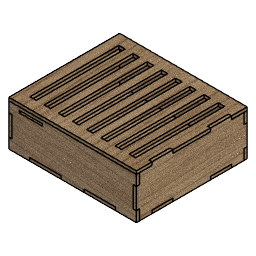
CAJA MADERA (Autodesk Fusion 360 design; units mm, degrees)
part number: 2026-06-24-23-30-10-522
part number: 2026-06-24-23-30-19-189
Autodesk Fusion 360 part; units mm, degrees
sketch "Boceto1" plane through (0, 0, 0) normal (0, 0, 1) x (1, 0, 0) in component "caja"
  line L0 (0, 0) -> (122, 0)
  line L1 (122, 0) -> (122, 106)
  line L2 (122, 106) -> (0, 106)
  line L3 (0, 106) -> (0, 0)
  dimension "d1" = 122
  dimension "d2" = 106
  constraint horizontal L0
  constraint vertical L1
  constraint horizontal L2
  constraint vertical L3
  constraint coincident L0.start L3.end
  measures "d1" distance of L0.start L0.end
  measures "d2" distance of L0.start L2.end
extrude "Extruir1" add sketch "Boceto1" along normal blind 3 makes body 1 in component "caja"
sketch "Boceto2" plane through (0, 0, 0) normal (0, -1, 0) x (1, 0, 0) in component "caja"
  line L0 (0, 0) -> (122, 0)
  line L1 (122, 0) -> (122, 3)
  line L2 (122, 3) -> (0, 3)
  line L3 (0, 3) -> (0, 0)
  line L4 (0, 0) -> (122, 0)
  line L5 (122, 0) -> (122, 40)
  line L6 (122, 40) -> (0, 40)
  line L7 (0, 40) -> (0, 0)
  line L8 (20, 0) -> (50, 0)
  line L9 (50, 0) -> (50, 3)
  line L10 (50, 3) -> (20, 3)
  line L11 (20, 3) -> (20, 0)
  line L12 (102, 0) -> (72, 0)
  line L13 (72, 0) -> (72, 3)
  line L14 (72, 3) -> (102, 3)
  line L15 (102, 3) -> (102, 0)
  line L16 (122, 30) -> (119, 30)
  line L17 (119, 30) -> (119, 10)
  line L18 (119, 10) -> (122, 10)
  line L19 (122, 10) -> (122, 30)
  line L20 (0, 30) -> (3, 30)
  line L21 (3, 30) -> (3, 10)
  line L22 (3, 10) -> (0, 10)
  line L23 (0, 10) -> (0, 30)
  point P0 (122, 20)
  point P1 (0, 20)
  dimension "d5" = 122
  dimension "d6" = 40
  dimension "d13" = 30
  dimension "d14" = 3
  dimension "d15" = 20
  dimension "d16" = 30
  dimension "d17" = 3
  dimension "d18" = 20
  dimension "d19" = 3
  dimension "d20" = 20
  dimension "d21" = 3
  dimension "d22" = 20
  constraint horizontal L4
  constraint vertical L5
  constraint horizontal L6
  constraint vertical L7
  constraint coincident L0.start L3.end
  constraint horizontal L8
  constraint vertical L9
  constraint horizontal L10
  constraint vertical L11
  constraint coincident L4 L8.start
  constraint horizontal L12
  constraint vertical L13
  constraint horizontal L14
  constraint vertical L15
  constraint coincident L4 L12.start
  constraint horizontal L16
  constraint vertical L17
  constraint horizontal L18
  constraint vertical L19
  constraint coincident L5 L16.start
  constraint midpoint L5 P0
  constraint midpoint L19 P0
  constraint horizontal L20
  constraint vertical L21
  constraint horizontal L22
  constraint vertical L23
  constraint coincident L7 L20.start
  constraint midpoint L7 P1
  constraint midpoint L23 P1
  measures "d5" distance of L0.start L0.end
  measures "d6" distance of L0.start L6.end
  measures "d13" distance of L8.start L8.end
  measures "d14" distance of L8.start L10.end
  measures "d15" distance of L0.start L8.start
  measures "d16" distance of L12.start L12.end
  measures "d17" distance of L12.start L14.end
  measures "d18" distance of L0.end L12.start
  measures "d19" distance of L16.start L16.end
  measures "d20" distance of L16.start L18.end
  measures "d21" distance of L20.start L20.end
  measures "d22" distance of L20.start L22.end
extrude "Extruir2" add sketch "Boceto2" against normal blind 3 separate body makes body 2 in component "caja"
sketch "Boceto3" plane through (122, 0, 0) normal (1, 0, 0) x (0, 1, 0) in component "caja"
  line L0 (0, 0) -> (106, 0)
  line L1 (106, 0) -> (106, 3)
  line L2 (106, 3) -> (0, 3)
  line L3 (0, 3) -> (0, 0)
  line L4 (0, 0) -> (106, 0)
  line L5 (106, 0) -> (106, 40)
  line L6 (106, 40) -> (0, 40)
  line L7 (0, 40) -> (0, 0)
  line L8 (15, 0) -> (35, 0)
  line L9 (35, 0) -> (35, 3)
  line L10 (35, 3) -> (15, 3)
  line L11 (15, 3) -> (15, 0)
  line L12 (91, 0) -> (71, 0)
  line L13 (71, 0) -> (71, 3)
  line L14 (71, 3) -> (91, 3)
  line L15 (91, 3) -> (91, 0)
  line L16 (15, 40) -> (35, 40)
  line L17 (35, 40) -> (35, 43)
  line L18 (35, 43) -> (15, 43)
  line L19 (15, 43) -> (15, 40)
  line L20 (71, 40) -> (91, 40)
  line L21 (91, 40) -> (91, 43)
  line L22 (91, 43) -> (71, 43)
  line L23 (71, 43) -> (71, 40)
  dimension "d9" = 106
  dimension "d10" = 40
  dimension "d25" = 20
  dimension "d26" = 3
  dimension "d27" = 15
  dimension "d28" = 20
  dimension "d29" = 3
  dimension "d30" = 15
  dimension "d45" = 20
  dimension "d46" = 3
  dimension "d47" = 20
  dimension "d48" = 3
  constraint horizontal L4
  constraint vertical L5
  constraint horizontal L6
  constraint vertical L7
  constraint coincident L0.start L3.end
  constraint horizontal L8
  constraint vertical L9
  constraint horizontal L10
  constraint vertical L11
  constraint coincident L0 L8.start
  constraint horizontal L12
  constraint vertical L13
  constraint horizontal L14
  constraint vertical L15
  constraint coincident L4 L12.start
  constraint horizontal L16
  constraint vertical L17
  constraint horizontal L18
  constraint vertical L19
  constraint coincident L6 L16.start
  constraint horizontal L20
  constraint vertical L21
  constraint horizontal L22
  constraint vertical L23
  constraint coincident L6 L20.start
  measures "d9" distance of L0.start L0.end
  measures "d10" distance of L0.start L6.end
  measures "d25" distance of L8.start L8.end
  measures "d26" distance of L8.start L10.end
  measures "d27" distance of L0.start L8.start
  measures "d28" distance of L12.start L12.end
  measures "d29" distance of L12.start L14.end
  measures "d30" distance of L0.end L12.start
  measures "d45" distance of L16.start L16.end
  measures "d46" distance of L16.start L18.end
  measures "d47" distance of L20.start L20.end
  measures "d48" distance of L20.start L22.end
extrude "Extruir3" add sketch "Boceto3" against normal blind 3 separate body contours L0 L2 L3 L4 L7 L11 | L0 L2 L4 L8 L9 L10 L11 | L2 L5 L6 L7 L10 L14 L16 L20 | L0 L2 L4 L9 L13 | L0 L2 L4 L12 L13 L14 L15 | L0 L1 L2 L4 L5 L15 makes body 3 in component "caja"
extrude "Extruir4" cut sketch "Boceto2" against normal blind 3 contours L0 L2 L4 L8 L9 L10 L11 | L7 L20 L21 L22 L23 | L0 L2 L4 L12 L13 L14 L15 | L5 L16 L17 L18 L19 bodies 2 in component "caja"
extrude "Extruir5" cut sketch "Boceto3" against normal blind 3 contours L0 L2 L4 L8 L9 L10 L11 | L0 L2 L4 L12 L13 L14 L15 bodies 3 in component "caja"
copy_body "CopiarPegarCuerpos1" bodies 2 makes body 4 in component "caja"
move_body "Desplazar1" bodies 4 to x (1, 0, 0) y (0, 1, 0) z (0, 0, 1) at (0, 126, 0) in component "caja"
copy_body "CopiarPegarCuerpos2" bodies 3 makes body 5 in component "caja"
move_body "Desplazar2" bodies 5 to x (1, 0, 0) y (0, 1, 0) z (0, 0, 1) at (-138, 0, 0) in component "caja"
move_body "Alinear1" bodies 5 to x (1, 0, 0) y (0, 1, 0) z (0, 0, 1) at (19, 0, 0) in component "caja"
move_body "Alinear2" bodies 4 to x (1, 0, 0) y (0, 1, 0) z (0, 0, 1) at (0, -23, 0) in component "caja"
combine "Combinar1" operation cut target body 1 tool bodies 2 5 4 3 keep tools in component "caja"
combine "Combinar2" operation cut target body 5 tool bodies 4 2 keep tools in component "caja"
combine "Combinar3" operation cut target body 3 tool bodies 2 4 keep tools in component "caja"
sketch "Boceto4" plane through (0, 0, 0) normal (0, -1, 0) x (1, 0, 0) in component "caja"
  line L0 (50, 3) -> (50, 0)
  line L1 (50, 0) -> (72, 0)
  line L2 (72, 0) -> (72, 3)
  line L3 (72, 3) -> (102, 3)
  line L4 (102, 3) -> (102, 0)
  line L5 (102, 0) -> (122, 0)
  line L6 (122, 0) -> (122, 10)
  line L7 (122, 10) -> (119, 10)
  line L8 (119, 10) -> (119, 30)
  line L9 (119, 30) -> (122, 30)
  line L10 (122, 30) -> (122, 40)
  line L11 (122, 40) -> (0, 40)
  line L12 (0, 40) -> (0, 30)
  line L13 (0, 30) -> (3, 30)
  line L14 (3, 30) -> (3, 10)
  line L15 (3, 10) -> (0, 10)
  line L16 (0, 10) -> (0, 0)
  line L17 (0, 0) -> (20, 0)
  line L18 (20, 0) -> (20, 3)
  line L19 (20, 3) -> (50, 3)
  line L20 (10.0905, 37.0618) -> (32.0905, 37.0618)
  line L21 (32.0905, 37.0618) -> (32.0905, 35.0618)
  line L22 (32.0905, 35.0618) -> (10.0905, 35.0618)
  line L23 (10.0905, 35.0618) -> (10.0905, 37.0618)
  dimension "d33" = 22
  dimension "d34" = 2
  constraint horizontal L20
  constraint vertical L21
  constraint horizontal L22
  constraint vertical L23
  measures "d33" distance of L20.start L20.end
  measures "d34" distance of L20.start L22.end
extrude "Extruir6" cut sketch "Boceto4" against normal blind 3 contours L20 L21 L22 L23 bodies 2 in component "caja"
sketch "Boceto5" plane through (0, 0, 0) normal (-1, 0, 0) x (0, -1, 0) in component "caja"
  line L0 (-3, 0) -> (-3, 10)
  line L1 (-3, 10) -> (0, 10)
  line L2 (0, 10) -> (0, 30)
  line L3 (0, 30) -> (-3, 30)
  line L4 (-3, 30) -> (-3, 40)
  line L5 (-3, 40) -> (-103, 40)
  line L6 (-103, 40) -> (-103, 30)
  line L7 (-103, 30) -> (-106, 30)
  line L8 (-106, 30) -> (-106, 10)
  line L9 (-106, 10) -> (-103, 10)
  line L10 (-103, 10) -> (-103, 0)
  line L11 (-103, 0) -> (-91, 0)
  line L12 (-91, 0) -> (-91, 3)
  line L13 (-91, 3) -> (-71, 3)
  line L14 (-71, 3) -> (-71, 0)
  line L15 (-71, 0) -> (-35, 0)
  line L16 (-35, 0) -> (-35, 3)
  line L17 (-35, 3) -> (-15, 3)
  line L18 (-15, 3) -> (-15, 0)
  line L19 (-15, 0) -> (-3, 0)
  line L20 (-12.0898, 37.3242) -> (-7.0898, 37.3242)
  line L21 (-7.0898, 37.3242) -> (-7.0898, 32.3242)
  line L22 (-7.0898, 32.3242) -> (-12.0898, 32.3242)
  line L23 (-12.0898, 32.3242) -> (-12.0898, 37.3242)
  dimension "d37" = 5
  dimension "d38" = 5
  constraint horizontal L20
  constraint vertical L21
  constraint horizontal L22
  constraint vertical L23
  measures "d37" distance of L20.start L20.end
  measures "d38" distance of L20.start L22.end
extrude "Extruir7" cut sketch "Boceto5" against normal blind 3 contours L20 L21 L22 L23 bodies 5 in component "caja"
sketch "Boceto8" plane through (0, 0, 40) normal (0, 0, 1) x (-1, 0, 0) in component "caja"
  line L0 (0, -103) -> (-122, -103)
  line L1 (-122, -103) -> (-122, -106)
  line L2 (-122, -106) -> (0, -106)
  line L3 (0, -106) -> (0, -103)
  line L4 (0, -106) -> (-122, -106)
  line L5 (-122, -106) -> (-122, 0)
  line L6 (-122, 0) -> (0, 0)
  line L7 (0, 0) -> (0, -106)
  line L8 (-10.0686, -95.2773) -> (-15.0686, -95.2773)
  line L9 (-15.0686, -95.2773) -> (-15.0686, -15.2773)
  line L10 (-15.0686, -15.2773) -> (-10.0686, -15.2773)
  line L11 (-10.0686, -15.2773) -> (-10.0686, -95.2773)
  dimension "d41" = 122
  dimension "d42" = 106
  dimension "d51" = 5
  dimension "d52" = 80
  constraint horizontal L4
  constraint vertical L5
  constraint horizontal L6
  constraint vertical L7
  constraint coincident L2.end L3.start
  constraint horizontal L8
  constraint vertical L9
  constraint horizontal L10
  constraint vertical L11
  measures "d41" distance of L2.end L1.end
  measures "d42" distance of L2.end L6.end
  measures "d51" distance of L8.start L8.end
  measures "d52" distance of L8.start L10.end
extrude "Extruir8" add sketch "Boceto8" along normal blind 3 separate body contours L0 L1 L2 L3 L4 L5 L7 | L0 L5 L6 L7 | L8 L9 L10 L11 makes body 6 in component "caja"
extrude "Extruir9" add sketch "Boceto3" against normal blind 3 contours L6 L16 L17 L18 L19 | L6 L20 L21 L22 L23 bodies 3 in component "caja"
combine "Combinar4" operation cut target body 6 tool bodies 3 keep tools in component "caja"
sketch "Boceto9" plane through (0, 0, 43) normal (0, 0, 1) x (-1, 0, 0) in component "caja"
  line L0 (-119, -91) -> (-122, -91)
  line L1 (-122, -91) -> (-122, -106)
  line L2 (-122, -106) -> (0, -106)
  line L3 (0, -106) -> (0, 0)
  line L4 (0, 0) -> (-122, 0)
  line L5 (-122, 0) -> (-122, -15)
  line L6 (-122, -15) -> (-119, -15)
  line L7 (-119, -15) -> (-119, -35)
  line L8 (-119, -35) -> (-122, -35)
  line L9 (-122, -35) -> (-122, -71)
  line L10 (-122, -71) -> (-119, -71)
  line L11 (-119, -71) -> (-119, -91)
  line L12 (-9.7376, -95.5293) -> (-15.7376, -95.5293)
  line L13 (-15.7376, -95.5293) -> (-15.7376, -10.5293)
  line L14 (-15.7376, -10.5293) -> (-9.7376, -10.5293)
  line L15 (-9.7376, -10.5293) -> (-9.7376, -95.5293)
  dimension "d53" = 6
  dimension "d54" = 85
  constraint horizontal L12
  constraint vertical L13
  constraint horizontal L14
  constraint vertical L15
  measures "d53" distance of L12.start L12.end
  measures "d54" distance of L12.start L14.end
extrude "Extruir10" cut sketch "Boceto9" against normal blind 3 contours L12 L13 L14 L15 bodies 6 in component "caja"
pattern_linear "Patrón R1" count 1 spacing 0 along (0, 0, 1) count 8 spacing 13.5714 along (1, 0, 0) of "Extruir10" in component "caja"
component "caja" placed x (1, 0, 0) y (0, 1, 0) z (0, 0, 1) at (0, 0, 0)
